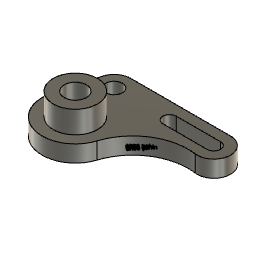
Model 15 (Autodesk Fusion 360 design; units mm, degrees)
Autodesk Fusion 360 part; units mm, degrees
sketch "Sketch1" plane through (0, 0, 0) normal (0, 0, 1) x (1, 0, 0)
  circle A0 centre (0, 0) radius 10
  circle A1 centre (0, 0) radius 20
  line L0 (0, 0) -> (85, 0) construction
  line L1 (85, 0) -> (85, 40) construction
  line L2 (85, 40) -> (45, 40) construction
  line L3 (45, 40) -> (45, 46) construction
  line L4 (85, 40) -> (85, 46) construction
  line L5 (45, 46) -> (85, 46)
  line L6 (45, 34) -> (85, 34)
  arc A2 (45, 46) -> (45, 34) centre (45, 40) ccw
  arc A3 (85, 34) -> (85, 46) centre (85, 40) ccw
  line L7 (45, 40) -> (-5, 40) construction
  circle A4 centre (-5, 40) radius 7.5
  line L8 (-5, 40) -> (-5, 55) construction
  line L9 (85, 40) -> (85, 55) construction
  line L10 (-5, 55) -> (85, 55)
  arc A5 (85, 24.817458) -> (28.570578, -9.149978) centre (76.188207, -24.39994) ccw
  line L11 (0, 0) -> (-30, 0) construction
  line L12 (-19.507658, 43.811543) -> (-29.015316, 7.623085)
  arc A6 (-5, 55) -> (-19.507658, 43.811543) centre (-5, 40) ccw
  arc A7 (-29.015316, 7.623085) -> (28.570578, -9.149978) centre (0, 0) ccw
  arc A8 (82.966509, 25.138475) -> (85, 55) centre (85, 40) ccw
  dimension "d1" = 20
  dimension "d2" = 40
  dimension "d3" = 60
  dimension "d4" = 85
  dimension "d5" = 40
  dimension "d6" = 12
  dimension "d8" = 40
  dimension "d9" = 12
  dimension "d10" = 50
  dimension "d11" = 15
  dimension "d12" = 30
  dimension "d14" = 100
  constraint coincident A0.centre A1.centre
  constraint concentric A0 A1
  constraint concentric A1 A7
  constraint horizontal L0
  constraint perpendicular L0 L1
  constraint coincident L1.end L2.start
  constraint perpendicular L1 L2
  constraint coincident L2.end L3.start
  constraint perpendicular L2 L3
  constraint perpendicular L2 L4
  constraint coincident L1 L6.end
  constraint tangent L6 A3
  constraint perpendicular L3 L7
  constraint coincident L7.end A4.centre
  constraint concentric A4 A6
  constraint perpendicular L7 L8
  constraint perpendicular L5 L9
  constraint tangent A5 A7
  constraint coincident L11.end A7
  constraint horizontal L11
  constraint tangent L12 A6
  constraint tangent L12 A7
  measures "d1" diameter of A0
  measures "d2" diameter of A1
  measures "d3" diameter of A7
  measures "d4" distance of A0.centre L0.end
  measures "d5" distance of L0.end L1.end
  measures "d6" diameter of A3
  measures "d8" distance of L1.end L2.end
  measures "d9" diameter of A2
  measures "d10" distance of L2.end L7.end
  measures "d11" diameter of A4
  measures "d12" diameter of A6
  measures "d14" diameter of A5
extrude "Extrude1" add sketch "Sketch1" along normal blind 15 contours L10 A5 L12 A6 A7 A8 picked at (17.105743, 31.25824)
extrude "Extrude2" add sketch "Sketch1" along normal blind 35 contours A1 picked at (16.554975, -1.490423)
ref_plane "WorkPlane1" through (37.885985, 7.73944, 8.074563) normal (0.766044, -0.642788, 0) x (-0.642788, -0.766044, 0)
sketch "Sketch2" plane through (37.885985, 7.73944, 8.074563) normal (0.766044, -0.642788, 0) x (-0.642788, -0.766044, 0)
  line L0 (14.782936, 3.28526) -> (-34.219154, 3.304929) construction
  line L1 (-34.219154, 3.304929) -> (-34.221012, -1.3215) construction
  line L2 (-34.221012, -1.3215) -> (14.781079, -1.34117) construction
  line L3 (14.781079, -1.34117) -> (14.782936, 3.28526) construction
  text T0 "enes şahin" font "Arial" height 3 align centre top in box 49.002095 x 4.62643 at (14.782936, 3.28526) x (-0.99999992, 0.0004014) y (-0.0004014, -0.99999992) spacing 1
extrude "Extrude3" add sketch "Sketch2" along normal blind 4 text T0
